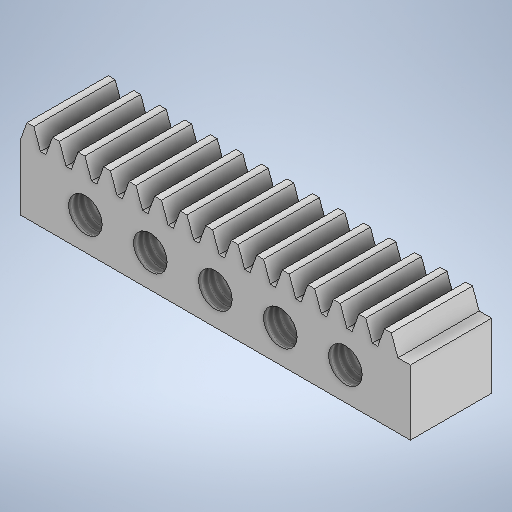
# Autodesk Inventor part: slizg
Saved by Autodesk Inventor 2025.2 (Build 292293000, 293)
## iProperties
Created: 2026-05-08
Part Number: slizg
Material: Ogólny
Document SubType Name: Modeling
Designer: muszy
Density: 1 g/cm^3
Appearance: Domyślna
Author: muszy
Autodesk Inventor part; units mm, degrees
ref_plane "YZ Plane" through (0, 0, 0) normal (1, 0, 0) x (0, 1, 0)
ref_plane "XZ Plane" through (0, 0, 0) normal (0, 1, 0) x (-1, 0, 0)
ref_plane "XY Plane" through (0, 0, 0) normal (0, 0, 1) x (1, 0, 0)
sketch "Szkic1" plane through (0, 0, 0) normal (0, 0, 1) x (1, 0, 0)
  line L0 (-24, -4) -> (24, -4)
  line L1 (24, -4) -> (24, 4)
  line L2 (24, 4) -> (-24, 4)
  line L3 (-24, 4) -> (-24, -4)
  line L4 (-24, -4) -> (24, 4) construction
  line L5 (24, -4) -> (-24, 4) construction
  point P0 (0, 0)
  dimension "d0" = 8
  dimension "d1" = 48
  constraints: 12 end point, 2 midpoint, 2 parallel, 1 horizontal, 1 perpendicular
  measures "d0" distance between parallel lines of L0 L2
  measures "d1" distance between parallel lines of L3 L1
extrude "Wyciągnięcie proste1" add sketch "Szkic1" along normal blind 10
sketch "Szkic2" plane through (0, 0, 10) normal (0, 0, 1) x (1, 0, 0)
  line L0 (0, 17.6829) -> (0, -21.534) construction
  line L1 (-24, 4) -> (-24, -4) projected
  point P0 (0, 0)
  point P1 (-16, 0)
  point P2 (-8, 0)
  point P3 (0, 0)
  point P4 (8, 0)
  point P5 (16, 0)
  dimension "d14" = 8
  dimension "d15" = 8
  dimension "d16" = 16
  constraints: 2 end point, 2 symmetric about line, 1 coincident, 1 vertical
  measures "d14" distance from line of L1 point (-16, 0)
  measures "d15" distance of point (-8, 0) point (-16, 0)
  measures "d16" diameter of point (-8, 0) L0
hole "Otwór1" at (-16, 0, 10) at (-8, 0, 10) at (0, 0, 10) at (8, 0, 10) at (16, 0, 10) direction (0, 0, -1) diameter 4.134 depth 7 tip angle 118 thread size "M5x0.8" class "6H" standard "ISO Metric profile"
sketch "Szkic4" plane through (0, 0, 10) normal (0, 0, 1) x (1, 0, 0)
  line L0 (-24, 4) -> (-23.1811, 6.25)
  line L1 (-23.1811, 6.25) -> (-22.3382, 6.25)
  line L2 (-22.3382, 6.25) -> (-21.5193, 4)
  line L3 (24, 4) -> (-24, 4) projected
  line L4 (-21.5193, 4) -> (-21.5193, 6.9311) construction
  line L5 (-24, 4) -> (-24, 7.0291) construction
  line L6 (-21.9742, 5.25) -> (-23.545, 5.25) construction
  point P0 (0, 0)
  dimension "d42" = 20
  dimension "d43" = 20
  dimension "d44" = 2.25
  dimension "d45" = 1.25
  dimension "d46" = 1.5708
  constraints: 12 end point, 3 point on line, 2 horizontal, 2 vertical
  measures "d42" angle of L0 L5
  measures "d43" angle of L2 L4
  measures "d44" distance between parallel lines of L3 L1
  measures "d45" distance between parallel lines of L3 L6
  measures "d46" distance of L6.start L6.end
extrude "Wyciągnięcie proste2" add sketch "Szkic4" against normal blind 10
pattern_linear "Szyk prostokątny2" count 15 spacing 3.1416 along (1, 0, 0) of "Wyciągnięcie proste2"
